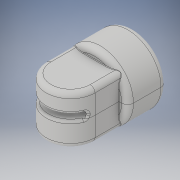
# Autodesk Inventor part: SimplifiedThigh040x
Saved by Autodesk Inventor 2018 (Build 220112000, 112)
## iProperties
Created: 2017-08-15
Part Number: SimplifiedThigh040x
Material: Generisch
Document SubType Name: Modeling
Designer: JochenAlt
Density: 1 g/cm^3
Appearance: Vorgabe
Mass: 57.7164 g
Surface Area: 269.653 cm^2
Volume: 57.7164 cm^3
Author: JochenAlt
Autodesk Inventor part; units mm, degrees
ref_plane "YZ Plane" through (0, 0, 0) normal (1, 0, 0) x (0, 1, 0)
ref_plane "Arbeitsebene2" through (0, 0, 0) normal (0, 0, 1) x (1, 0, 0)
sketch "Skizze Herkulex 040x" plane through (0, 0, 0) normal (0, 0, 1) x (1, 0, 0)
  line L0 (0, -49.2432) -> (0, 42.9739) construction
  line L1 (-28.937, 0) -> (28.937, 0) construction
  line L2 (14.8, 28.3) -> (-14.8, 28.3)
  line L3 (-17.8, 25.3) -> (-17.8, -22.3)
  line L4 (-11.8, -28.3) -> (11.8, -28.3)
  line L5 (17.8, -22.3) -> (17.8, 25.3)
  line L6 (17.8, 28.3) -> (-17.8, -28.3) construction
  line L7 (-17.8, 28.3) -> (17.8, -28.3) construction
  arc A0 (-17.8, -22.3) -> (-11.8, -28.3) centre (-11.8, -22.3) ccw
  arc A1 (11.8, -28.3) -> (17.8, -22.3) centre (11.8, -22.3) ccw
  arc A2 (17.8, 25.3) -> (14.8, 28.3) centre (14.8, 25.3) ccw
  arc A3 (-14.8, 28.3) -> (-17.8, 25.3) centre (-14.8, 25.3) ccw
  line L8 (8.5, 21.2) -> (-8.5, 21.2)
  line L9 (-11.5, 18.2) -> (-11.5, -25.3)
  line L10 (-8.5, -28.3) -> (8.5, -28.3)
  line L11 (11.5, -25.3) -> (11.5, 18.2)
  line L12 (11.5, 21.2) -> (-11.5, -28.3) construction
  line L13 (-11.5, 21.2) -> (11.5, -28.3) construction
  arc A4 (-11.5, -25.3) -> (-8.5, -28.3) centre (-8.5, -25.3) ccw
  arc A5 (-8.5, 21.2) -> (-11.5, 18.2) centre (-8.5, 18.2) ccw
  arc A6 (11.5, 18.2) -> (8.5, 21.2) centre (8.5, 18.2) ccw
  arc A7 (8.5, -28.3) -> (11.5, -25.3) centre (8.5, -25.3) ccw
  circle A8 centre (0, -15.4) radius 12.75
  circle A9 centre (-13.5, 23.5) radius 1.3
  circle A10 centre (13.5, 23.5) radius 1.3
  line L14 (-13.5, -22.4) -> (13.5, -22.4) construction
  line L15 (13.5, -22.4) -> (13.5, 23.5) construction
  line L16 (13.5, 23.5) -> (-13.5, 23.5) construction
  line L17 (-13.5, 23.5) -> (-13.5, -22.4) construction
  line L18 (5.5, -8.75) -> (-5.5, -8.75) construction
  line L19 (5.5, -18.5) -> (-5.5, -18.5)
  line L20 (-5.5, 1) -> (5.5, 1)
  arc A11 (5.5, -18.5) -> (5.5, 1) centre (5.5, -8.75) ccw
  arc A12 (-5.5, 1) -> (-5.5, -18.5) centre (-5.5, -8.75) ccw
  circle A13 centre (0, -15.4) radius 4
  line L21 (-20.6693, 29.8) -> (20.6693, 29.8)
  line L22 (-20.6693, 29.8) -> (-20.6693, -15.4)
  line L23 (20.6693, -15.4) -> (20.6693, 29.8)
  arc A14 (-20.6693, -15.4) -> (20.6693, -15.4) centre (0, -15.4) ccw
  circle A15 centre (-13.5, 23.5) radius 2.5
  circle A16 centre (13.5, 23.5) radius 2.5
  arc A17 (14, -23.6) -> (14, -21.2) centre (14, -22.4) ccw construction
  arc A18 (14, -21.2) -> (14, -23.6) centre (14, -22.4) ccw construction
  arc A19 (-14, -21.2) -> (-14, -23.6) centre (-14, -22.4) ccw construction
  arc A20 (-14, -23.6) -> (-14, -21.2) centre (-14, -22.4) ccw construction
  circle A21 centre (14, -22.4) radius 1
  circle A22 centre (-14, -22.4) radius 1
  circle A23 centre (0, 15) radius 10
  point P0 (0, 0)
  point P1 (0, -3.55)
  point P2 (0, -8.75)
  dimension "d115" = 35.6
  dimension "d116" = 56.6
  dimension "d117" = 6
  dimension "d118" = 49.5
  dimension "d119" = 23
  dimension "d120" = 3
  dimension "d121" = 25.5
  dimension "d122" = 15.4
  dimension "d124" = 2.6
  dimension "d125" = 2.6
  dimension "d128" = 45.9
  dimension "d129" = 7
  dimension "d130" = 19.5
  dimension "d131" = 30.5
  dimension "d132" = 8
  dimension "d163" = 1.5
  dimension "d167" = 1
  dimension "d169" = 5
  dimension "d170" = 5
  dimension "d171" = 27
  dimension "d219" = 2
  dimension "d220" = 2
  dimension "d221" = 3
  dimension "d222" = 3
  dimension "d223" = 3
  dimension "d224" = 1
  dimension "d225" = 20
  dimension "d226" = 15
  constraints: 46 end point, 30 point on circle, 24 centre point, 22 point on line, 22 tangent, 8 parallel, 6 midpoint, 5 coincident, 4 perpendicular, 3 concentric, 3 horizontal, 2 equal radius, 1 collinear, 1 vertical, 13 other
  measures "d115" distance of L7.end L6.end
  measures "d116" distance of L6.end L7.start
  measures "d117" radius of A0
  measures "d118" distance between parallel lines of L8 L10
  measures "d119" distance between parallel lines of L11 L9
  measures "d120" radius of A4
  measures "d121" diameter of A8
  measures "d122" distance of A8.centre point (0, 0)
  measures "d124" diameter of A9
  measures "d125" diameter of A10
  measures "d128" distance between parallel lines of L16 L14
  measures "d129" distance from line of A8.centre L14
  measures "d130" distance between parallel lines of L20 L19
  measures "d132" diameter of A13
  measures "d163" distance between parallel lines of L21 L2
  measures "d169" diameter of A15
  measures "d170" diameter of A16
  measures "d171" distance between parallel lines of L15 L17
  measures "d219" diameter of A21
  measures "d220" diameter of A22
  measures "d221" radius of A2
  measures "d222" radius of A3
  measures "d223" radius of A6
  measures "d224" distance between parallel lines of L1 L20
  measures "d225" diameter of A23
  measures "d226" distance from line of L1 A23.centre
extrude "Extrusion1" [suppressed]
fillet "Rundung11" [suppressed]
extrude "Extrusion2" [suppressed]
extrude "Extrusion3" [suppressed]
extrude "Extrusion4" [suppressed]
extrude "Extrusion5" add sketch "Skizze Herkulex 040x" against normal blind 36.4 and the other way blind 4.6 separate body contours A2 L5 A1 L4 A7 L11 A8 A11 A6 L8 A23 A5 L9 A12 A4 A0 L3 A3 L2 | L4 A4 L9 A8 L11 A7 | A8 L9 A12 L19 A13 A11 L11 | L11 A11 A8 | A8 A12 L9 | A11 L19 A13 A12 L9 A8 L11 | L11 A8 A11 | A12 A8 L9 | A12 L9 A8 | A8 L9 A12 L20 A11 L11 | L11 A11 A8 | L9 A5 L8 A23 A6 L11 A11 L20 A12 | A13 L19 | L19 A13 | A23 L8 | L8 A23 | A9 | A10 | L21 L23 A14 L22 | A15 | A16 | A21 | A22
sketch "Skizze4" plane through (-23.6693, 29.8, -36.4) normal (0, 1, 0) x (1, 0, 0)
  circle A0 centre (23.6693, -20.5) radius 28
  line L0 (44.3386, -41) -> (44.3386, 0) construction
  line L1 (3, 0) -> (44.3386, 0) construction
  line L2 (3, 0) -> (3, -41) construction
  line L3 (44.3386, -41) -> (3, -41) construction
  line L4 (3, -41) -> (44.3386, -41) construction
  line L5 (44.3386, 0) -> (3, 0) construction
  line L6 (3, -41) -> (44.3386, 0) construction
  line L7 (3, -41) -> (3, 0) construction
  line L8 (44.3386, -41) -> (3, 0) construction
  dimension "d168" = 56
  constraints: 4 end point, 1 centre point, 1 midpoint
  measures "d168" diameter of A0
sketch "Skizze Lagerflansch" plane through (0, -16.4396, 4.6) normal (0, 0, 1) x (1, 0, 0)
  circle A0 centre (0, 1.0239) radius 4
  circle A1 centre (0, 1.0239) radius 3.4
  point P0 (0, 16.4396)
  dimension "d73" = 8
  dimension "d76" = 6.8
  constraints: 2 centre point, 1 coincident
  measures "d73" diameter of A0
  measures "d76" diameter of A1
extrude "Extrusion Lagerflansch" [suppressed]
extrude "Extrusion Lagerachse" [suppressed]
chamfer "Fase8" [suppressed]
fillet "Rundung3" radius 4.1 6 edges at (0, -36.0693, -36.4) (20.6693, 7.2, -36.4) (-20.6693, 7.2, -36.4) (0, -36.0693, 4.6) (20.6693, 7.2, 4.6) (-20.6693, 7.2, 4.6)
extrude "Extrusion6" add sketch "Skizze4" along normal blind 8.3 and the other way blind 25
feature "Kombinieren1" [suppressed]
ref_plane "Trennfläche" through (0, 29.8, -15.9) normal (0, 0, 1) x (1, 0, 0)
sketch "Skizze16" plane through (0, 0.1, -15.9) normal (0, 0, 1) x (1, 0, 0)
  line L0 (33.5581, -20.9355) -> (-28.6036, -20.9355)
  line L1 (-28.6036, -20.9355) -> (-28.6036, -48.1191)
  line L2 (-28.6036, -48.1191) -> (33.5581, -48.1191)
  line L3 (33.5581, -48.1191) -> (33.5581, -20.9355)
  line L4 (-28.6036, -63.6829) -> (-28.6036, 45.2638) construction
  line L5 (-41.036, -0.1) -> (45.9904, -0.1) construction
  point P0 (0, -0.1)
  point P1 (-28.6036, 45.2638)
  point P2 (-20.6693, -20.9355)
  constraints: 8 end point, 2 parallel, 1 horizontal, 1 perpendicular, 1 point on line, 1 vertical, 3 other
extrude "Extrusion20" cut sketch "Skizze16" along normal blind 5
fillet "Rundung9" radius 2 2 edges at (0, -20.8355, -10.9) (0, -20.8355, -15.9)
fillet "Rundung10" radius 2 2 edges at (0, -36.0693, -15.9) (0, -36.0693, -10.9)
fillet "Rundung4" radius 5 1 edges at (-28, 4.8, -15.9)
fillet "Rundung5" radius 0.5 17 edges at (-20.6693, 5.0627, -29.2383) (-19.4629, 7.4495, -35.2047) (-13.5906, 5.0615, -36.4) (0, 4.8, -36.4) (13.5906, 5.0615, -36.4) (19.4659, 7.4495, -35.2016) (20.6693, 5.0627, -29.2383) (20.6693, 4.8, -15.9) (20.6693, 5.0627, -2.5618) (20.6693, 6.1203, 0.5) (19.4625, 7.4495, 3.405) (13.5906, 5.0615, 4.6) (0, 4.8, 4.6) (-13.5906, 5.0615, 4.6) (-19.4656, 7.4495, 3.402) (-20.6693, 5.0627, -2.5618) (-20.6693, 4.8, -15.9)
sketch "Skizze5" plane through (0, 38.1, -15.9) normal (0, 1, 0) x (1, 0, 0)
  circle A0 centre (0, 0) radius 21
  point P0 (0, -15.9)
  dimension "d54" = 42
  constraints: 1 centre point
  measures "d54" diameter of A0
extrude "Extrusion7" [suppressed]
sketch "Skizze6" plane through (0, 36.9, -15.9) normal (0, 1, 0) x (1, 0, 0)
  circle A0 centre (0, 0) radius 22.4
  point P0 (0, -15.9)
  dimension "d57" = 44.8
  constraints: 1 centre point
  measures "d57" diameter of A0
extrude "Extrusion8" [suppressed]
sketch "Skizze7" plane through (0, 31.8, -15.9) normal (0, 1, 0) x (1, 0, 0)
  circle A0 centre (0, 0) radius 20.5
  point P0 (0, -15.9)
  dimension "d60" = 41
  constraints: 1 centre point
  measures "d60" diameter of A0
extrude "Extrusion9" [suppressed]
sketch "Skizze8" plane through (0, 30.3, -15.9) normal (0, 1, 0) x (1, 0, 0)
  line L0 (-39.2, -15.9) -> (39.2, -15.9) construction
  line L1 (0, 39.2) -> (0, -39.2) construction
  line L2 (10.6207, 9.1215) -> (10.6207, -9.1215)
  arc A0 (10.6207, 9.1215) -> (-10.6207, 9.1215) centre (0, 0) ccw
  arc A1 (-10.6207, -9.1215) -> (10.6207, -9.1215) centre (0, 0) ccw
  line L3 (-10.6207, 9.1215) -> (-10.6207, -9.1215)
  circle A2 centre (0, 0) radius 20.5 projected
  line L4 (10.6207, -9.1215) -> (-10.6207, 9.1215) construction
  line L5 (-10.6207, -9.1215) -> (10.6207, 9.1215) construction
  point P0 (0, -15.9)
  point P1 (0, 0)
  dimension "d237" = 14
  dimension "d238" = 14
  constraints: 8 end point, 5 point on circle, 2 centre point, 2 midpoint, 1 concentric, 1 vertical
  measures "d237" radius of A0
  measures "d238" radius of A1
extrude "Extrusion10" [suppressed]
sketch "Skizze9" plane through (0, 31.8, -15.9) normal (0, 1, 0) x (1, 0, 0)
  circle A0 centre (0, 0) radius 8
  point P0 (0, -15.9)
  dimension "d67" = 16
  constraints: 1 centre point
  measures "d67" diameter of A0
extrude "Extrusion11" [suppressed]
sketch "Skizze22" plane through (0, 29.8, -15.9) normal (0, 0, 1) x (1, 0, 0)
  line L0 (0, 0.7) -> (14, 0.7)
  arc A0 (18.5, -3.8) -> (14, 0.7) centre (14, -3.8) ccw
  line L1 (-17.8, -4.5) -> (-18.612, -4.5)
  line L2 (-17.8, -4.5) -> (-17.612, -3.2035)
  line L3 (-16.8141, -54.4699) -> (-17.8141, -54.4699)
  line L4 (-18.612, -10.1) -> (0, -10.1)
  line L5 (8.5, -58.1) -> (-8.5, -58.1) projected
  line L6 (-18.5, -72.2017) -> (-18.5, -21.1)
  line L7 (-18.5, -72.2017) -> (18.5, -72.2017)
  line L8 (0, 0.7) -> (0, -10.1)
  line L9 (-24.5, -21.1) -> (-24.5, -10.1)
  line L10 (18.5, -3.8) -> (18.5, -10.1)
  line L11 (18.5, -21.1) -> (18.5, -72.2017)
  line L12 (0, -86.9684) -> (0, 16.3987) construction
  line L13 (-18.5, -21.1) -> (-24.5, -21.1)
  line L14 (-24.5, -10.1) -> (0, -10.1)
  line L15 (18.5, -21.1) -> (-18.5, -21.1)
  line L16 (18.5, -10.1) -> (0, -10.1)
  line L17 (18.5, -21.1) -> (18.5, -10.1)
  line L18 (20.6693, -45.2) -> (20.6693, -23.9964) projected
  line L19 (-20.5, 0.5) -> (20.5, 0.5) construction
  line L20 (17.8, -4.5) -> (17.8, -52.1) construction
  line L21 (17.8, -52.1) -> (17.8, -4.5) projected
  line L22 (17.8, -10.1) -> (17.8, -21.1)
  line L23 (14.8, -1.5) -> (-14.8, -1.5) construction
  point P0 (-17.8, -52.1)
  dimension "d249" = 6
  dimension "d251" = 0.7
  dimension "d273" = 2.2
  constraints: 34 end point, 6 horizontal, 5 point on line, 3 tangent, 2 collinear, 2 perpendicular, 2 point on circle, 1 centre point, 1 parallel, 1 other
  measures "d249" distance between parallel lines of L9 L6
  measures "d251" distance between parallel lines of L11 L20
  measures "d273" distance between parallel lines of L23 L0
extrude "Extrusion24" cut sketch "Skizze22" along normal blind 5
extrude "Extrusion26" cut sketch "Skizze22" against normal blind 7 contours L16 L21 L15 L13 L9 L14 L4
fillet "Rundung6" radius 5 1 edges at (-28, 38.1, -15.9)
sketch "Skizze14" plane through (-16.1, 28.3, 0) normal (0, -1, 0) x (1, 0, 0)
  line L0 (7.1, -6.9) -> (25.1, -6.9)
  line L1 (25.1, -6.9) -> (25.1, -24.9)
  line L2 (25.1, -24.9) -> (7.1, -24.9)
  line L3 (7.1, -24.9) -> (7.1, -6.9)
  line L4 (7.1, -6.9) -> (25.1, -24.9) construction
  line L5 (25.1, -6.9) -> (7.1, -24.9) construction
  line L6 (32.4654, -8.2) -> (-2.5346, -8.2)
  line L7 (-2.5346, -8.2) -> (-2.5346, -18.2)
  line L8 (-2.5346, -18.2) -> (32.4654, -18.2)
  line L9 (32.4654, -18.2) -> (32.4654, -8.2)
  line L10 (32.4654, -8.2) -> (-2.5346, -18.2) construction
  line L11 (-2.5346, -8.2) -> (32.4654, -18.2) construction
  circle A0 centre (16.1, -15.9) radius 28 construction
  point P0 (16.1, 0)
  point P1 (14.9654, -13.2)
  point P2 (16, 0)
  point P3 (16, 0)
  point P4 (16, 0)
  dimension "d98" = 18
  dimension "d99" = 18
  dimension "d102" = 10
  dimension "d103" = 8.2
  dimension "d104" = 35
  constraints: 24 end point, 4 midpoint, 4 parallel, 2 horizontal, 2 perpendicular, 1 coincident
  measures "d98" distance of L1.end L2.end
  measures "d99" distance of L0.end L1.end
  measures "d102" distance between parallel lines of L6 L8
  measures "d103" distance from line of point (16.1, 0) L6
  measures "d104" distance between parallel lines of L7 L9
extrude "Extrusion19" [suppressed]
extrude "Extrusion16" [suppressed]
ref_plane "Arbeitsebene7" through (-14.8, 27.3, -33.9) normal (0, 0, 1) x (1, 0, 0)
extrude "Extrusion17" [suppressed]
ref_plane "Arbeitsebene8" through (14.8, 27.3, 2) normal (0, 0, -1) x (-1, 0, 0)
extrude "Extrusion18" [suppressed]
chamfer "Fase18" [suppressed]
fillet "Rundung20" [suppressed]
fillet "Rundung21" [suppressed]
split body "Trennen3" result two bodies by plane through (0, 29.8, -15.9) normal (0, 0, 1) first body at (-6.1667, -12.3237, -10.4)
